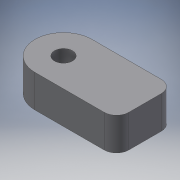
# Autodesk Inventor part: Motor Axle Fitting Test
Saved by Autodesk Inventor 2020 (Build 240168000, 168)
## iProperties
Created: 2020-02-06
Part Number: Motor Axle Fitting Test
Material: Generic
Document SubType Name: Modeling
Designer: Wes
Density: 1 g/cm^3
Appearance: Default
Author: Wes
Autodesk Inventor part; units mm, degrees
ref_plane "YZ Plane" through (0, 0, 0) normal (1, 0, 0) x (0, 1, 0)
ref_plane "XZ Plane" through (0, 0, 0) normal (0, 1, 0) x (-1, 0, 0)
ref_plane "XY Plane" through (0, 0, 0) normal (0, 0, 1) x (1, 0, 0)
sketch "Sketch1 - base" plane through (0, 0, 0) normal (0, 0, 1) x (1, 0, 0)
  circle A0 centre (0, 0) radius 3.5
  line L0 (-3.5, 0) -> (-3.5, 10)
  line L1 (-3.5, 10) -> (3.5, 10)
  line L2 (3.5, 10) -> (3.5, 0)
  dimension "d0" = 7
  dimension "d1" = 10
  constraints: 6 end point, 2 point on circle, 1 centre point, 1 horizontal, 1 perpendicular, 1 tangent, 1 vertical
  measures "d0" diameter of A0
  measures "d1" distance of L0.start L0.end
extrude "Extrusion1" add sketch "Sketch1 - base" along normal blind 4
sketch "Sketch2 - axle_hole" plane through (0, 0, 0) normal (0, 0, -1) x (-1, 0, 0)
  circle A0 centre (0, 0) radius 2.275
  arc A1 (-2.1959, 0.5948) -> (-2.275, 0) centre (-2.256, 0.3001) ccw
  line L0 (-2.256, 0.3001) -> (-2.5544, 0.3398) construction
  arc A2 (-2.2722, -0.1129) -> (-2.1637, -0.703) centre (-2.2383, -0.4117) ccw
  arc A3 (-2.1261, -0.8095) -> (-1.8405, -1.3372) centre (-2.0015, -1.0832) ccw
  arc A4 (-1.7719, -1.4269) -> (-1.3372, -1.8405) centre (-1.5688, -1.6487) ccw
  arc A5 (-1.2442, -1.9046) -> (-0.703, -2.1637) centre (-0.9826, -2.0528) ccw
  arc A6 (-0.5948, -2.1959) -> (0, -2.275) centre (-0.3001, -2.256) ccw
  arc A7 (0.1129, -2.2722) -> (0.703, -2.1637) centre (0.4117, -2.2383) ccw
  arc A8 (0.8095, -2.1261) -> (1.3372, -1.8405) centre (1.0832, -2.0015) ccw
  arc A9 (1.4269, -1.7719) -> (1.8405, -1.3372) centre (1.6487, -1.5688) ccw
  arc A10 (1.9046, -1.2442) -> (2.1637, -0.703) centre (2.0528, -0.9826) ccw
  arc A11 (2.1959, -0.5948) -> (2.275, 0) centre (2.256, -0.3001) ccw
  arc A12 (2.2722, 0.1129) -> (2.1637, 0.703) centre (2.2383, 0.4117) ccw
  arc A13 (2.1261, 0.8095) -> (1.8405, 1.3372) centre (2.0015, 1.0832) ccw
  arc A14 (1.7719, 1.4269) -> (1.3372, 1.8405) centre (1.5688, 1.6487) ccw
  arc A15 (1.2442, 1.9046) -> (0.703, 2.1637) centre (0.9826, 2.0528) ccw
  arc A16 (0.5948, 2.1959) -> (0, 2.275) centre (0.3001, 2.256) ccw
  arc A17 (-0.1129, 2.2722) -> (-0.703, 2.1637) centre (-0.4117, 2.2383) ccw
  arc A18 (-0.8095, 2.1261) -> (-1.3372, 1.8405) centre (-1.0832, 2.0015) ccw
  arc A19 (-1.4269, 1.7719) -> (-1.8405, 1.3372) centre (-1.6487, 1.5688) ccw
  arc A20 (-1.9046, 1.2442) -> (-2.1637, 0.703) centre (-2.0528, 0.9826) ccw
  point P0 (-2.2722, -0.1129)
  point P1 (-2.1261, -0.8095)
  point P2 (-1.8405, -1.3372)
  point P3 (-1.3372, -1.8405)
  point P4 (-1.2442, -1.9046)
  point P5 (-0.5948, -2.1959)
  point P6 (0, -2.275)
  point P7 (0.1129, -2.2722)
  point P8 (0.8095, -2.1261)
  point P9 (1.3372, -1.8405)
  point P10 (1.4269, -1.7719)
  point P11 (1.8405, -1.3372)
  point P12 (1.9046, -1.2442)
  point P13 (2.1637, -0.703)
  point P14 (2.1959, -0.5948)
  point P15 (2.275, 0)
  point P16 (2.2722, 0.1129)
  point P17 (2.1637, 0.703)
  point P18 (2.1261, 0.8095)
  point P19 (1.8405, 1.3372)
  point P20 (1.7719, 1.4269)
  point P21 (1.3372, 1.8405)
  point P22 (1.2442, 1.9046)
  point P23 (0.703, 2.1637)
  point P24 (0.5948, 2.1959)
  point P25 (0, 2.275)
  point P26 (-0.1129, 2.2722)
  point P27 (-0.703, 2.1637)
  point P28 (-0.8095, 2.1261)
  point P29 (-1.3372, 1.8405)
  point P30 (-1.4269, 1.7719)
  point P31 (-1.8405, 1.3372)
  point P32 (-1.9046, 1.2442)
  point P33 (-2.1637, 0.703)
  dimension "d4" = 4.55
  dimension "d16" = 0.6
  dimension "d17" = 0.301
  dimension "d20" = 360
  constraints: 40 point on circle, 20 centre point, 2 end point, 1 coincident, 85 other
  measures "d16" distance of A1.end A1.start
  measures "d17" distance of L0.start L0.end
extrude "Extrusion2" cut sketch "Sketch2 - axle_hole" against normal blind 2
sketch "Sketch3 - screw_hole" plane through (0, 0, 0) normal (0, 0, -1) x (-1, 0, 0)
  circle A0 centre (0, 0) radius 1.1
  dimension "d12" = 2.2
  constraints: 1 centre point, 1 coincident
  measures "d12" diameter of A0
extrude "Extrusion3" cut sketch "Sketch3 - screw_hole" against normal blind 4
fillet "Fillet1" radius 1.5 2 edges at (3.5, 10, 2) (-3.5, 10, 2)
body "Solid1"
